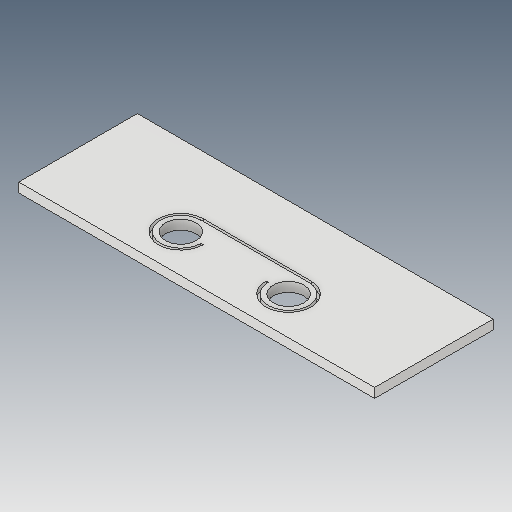
# Autodesk Inventor part: 2ureactor TorusTapa1
Saved by Autodesk Inventor 2018 (Build 220112000, 112)
## iProperties
Created: 2018-10-26
Part Number: 2ureactor TorusTapa1
Material: PPS Plastic
Document SubType Name: Modeling
Designer: mj.noguera10
Density: 1.637 g/cm^3
Appearance: Smooth - White
Author: mj.noguera10
Autodesk Inventor part; units mm, degrees
ref_plane "YZ Plane" through (0, 0, 0) normal (1, 0, 0) x (0, 1, 0)
ref_plane "XZ Plane" through (0, 0, 0) normal (0, 1, 0) x (-1, 0, 0)
ref_plane "XY Plane" through (0, 0, 0) normal (0, 0, 1) x (1, 0, 0)
sketch "Sombreado_1" plane through (0, 0, 0) normal (0, 0, 1) x (1, 0, 0)
  point P0 (0, 0)
sketch "Sombreado_2" plane through (0, 0, 0) normal (0, 0, 1) x (1, 0, 0)
  point P0 (0, 0)
sketch "Sombreado_3" plane through (0, 0, 0) normal (0, 0, 1) x (1, 0, 0)
  point P0 (0, 0)
sketch "Boceto1" plane through (0, 0, 0) normal (0, 1, 0) x (-1, 0, 0)
  line L0 (30.3882, 1.25) -> (30.8882, 1.25)
  line L1 (0, -6.75) -> (75, -6.75)
  line L2 (75, -6.75) -> (75, 18.25)
  line L3 (75, 18.25) -> (0, 18.25)
  line L4 (0, 18.25) -> (0, -6.75)
  arc A0 (21.3882, 1.25) -> (30.8882, 1.25) centre (26.1382, 1.25) ccw
  arc A1 (21.8882, 1.25) -> (30.3882, 1.25) centre (26.1382, 1.25) ccw
  line L5 (21.3882, 1.25) -> (21.8882, 1.25)
  line L6 (1.8, 2.5) -> (5.3, 2.5)
  line L7 (1.8, 2.5) -> (1.8, 3)
  line L8 (1.8, 3) -> (1, 3)
  line L9 (1, 3) -> (1, 2.5)
  line L10 (1, 0) -> (0, 0)
  line L11 (1, 0) -> (1, -0.5)
  line L12 (1, -0.5) -> (1.8, -0.5)
  line L13 (1.8, -0.5) -> (1.8, 0)
  line L14 (5.3, 0) -> (1.8, 0)
  line L15 (0, 2.5) -> (1, 2.5)
  line L16 (1.8, 11.5) -> (5.3, 11.5)
  line L17 (5.3, 9) -> (1.8, 9)
  line L18 (1, 9) -> (0, 9)
  line L19 (0, 11.5) -> (1, 11.5)
  line L20 (1.8, 11.5) -> (1.8, 12)
  line L21 (1.8, 12) -> (1, 12)
  line L22 (1, 12) -> (1, 11.5)
  line L23 (1, 9) -> (1, 8.5)
  line L24 (1, 8.5) -> (1.8, 8.5)
  line L25 (1.8, 8.5) -> (1.8, 9)
  line L26 (44.6082, 1.25) -> (44.1082, 1.25)
  arc A2 (44.1082, 1.25) -> (53.6082, 1.25) centre (48.8582, 1.25) ccw
  arc A3 (44.6082, 1.25) -> (53.1082, 1.25) centre (48.8582, 1.25) ccw
  line L27 (53.6082, 1.25) -> (53.1082, 1.25)
  line L28 (73.1964, 2.5) -> (69.6964, 2.5)
  line L29 (69.6964, 0) -> (73.1964, 0)
  line L30 (73.9964, 0) -> (74.9964, 0)
  line L31 (74.9964, 2.5) -> (73.9964, 2.5)
  line L32 (73.1964, 2.5) -> (73.1964, 3)
  line L33 (73.1964, 3) -> (73.9964, 3)
  line L34 (73.9964, 3) -> (73.9964, 2.5)
  line L35 (73.9964, 0) -> (73.9964, -0.5)
  line L36 (73.9964, -0.5) -> (73.1964, -0.5)
  line L37 (73.1964, -0.5) -> (73.1964, 0)
  line L38 (73.1964, 11.5) -> (69.6964, 11.5)
  line L39 (69.6964, 9) -> (73.1964, 9)
  line L40 (73.9964, 9) -> (74.9964, 9)
  line L41 (74.9964, 11.5) -> (73.9964, 11.5)
  line L42 (73.1964, 11.5) -> (73.1964, 12)
  line L43 (73.1964, 12) -> (73.9964, 12)
  line L44 (73.9964, 12) -> (73.9964, 11.5)
  line L45 (73.9964, 9) -> (73.9964, 8.5)
  line L46 (73.9964, 8.5) -> (73.1964, 8.5)
  line L47 (73.1964, 8.5) -> (73.1964, 9)
  line L48 (75, 18.25) -> (75, 43.25)
  line L49 (75, 43.25) -> (0, 43.25)
  line L50 (0, 43.25) -> (0, 18.25)
  line L51 (5.3, 11.5) -> (5.3, 9)
  line L52 (5.3, 2.5) -> (5.3, 0)
  line L53 (69.6964, 11.5) -> (69.6964, 9)
  line L54 (69.6964, 2.5) -> (69.6964, 0)
  circle A4 centre (26.1382, 1.25) radius 3.25
  circle A5 centre (48.8582, 1.25) radius 3.25
  circle A6 centre (26.1382, 26.25) radius 3.25
  circle A7 centre (48.8582, 26.25) radius 3.25
  line L55 (75, 43.25) -> (75, 68.25)
  line L56 (75, 68.25) -> (0, 68.25)
  line L57 (0, 68.25) -> (0, 43.25)
  circle A8 centre (26.1382, 51.25) radius 3.25
  circle A9 centre (48.8582, 51.25) radius 3.25
  point P0 (0, 0)
  constraints: 116 end point, 10 centre point, 8 point on circle
sketch "Boceto3" plane through (0, 0, 0) normal (0, 1, 0) x (-1, 0, 0)
  line L0 (0, 0) -> (-75, 0)
  line L1 (-75, 0) -> (-75, -25)
  line L2 (-75, -25) -> (0, -25)
  line L3 (0, -25) -> (0, 0)
  line L4 (0, 0) -> (-75, 0)
  line L5 (-75, 0) -> (-75, -25)
  line L6 (-75, -25) -> (0, -25)
  line L7 (0, -25) -> (0, 0)
  dimension "d4" = 75
  dimension "d5" = 25
  dimension "d6" = 75
  dimension "d7" = 25
  constraints: 16 end point, 4 parallel, 2 horizontal, 2 perpendicular
  measures "d4" distance of L2.end L1.end
  measures "d5" distance of L1.end L1.start
  measures "d6" distance of L6.end L5.end
  measures "d7" distance of L5.end L5.start
extrude "Extrusión1" add sketch "Boceto3" along normal blind 2
sketch "Boceto4" plane through (0, 2, 0) normal (0, 1, 0) x (1, 0, 0)
  circle A0 centre (26.1418, 8) radius 3.25
  line L0 (0, 0) -> (75, 0) projected
  line L1 (75, 25) -> (0, 25) projected
  circle A1 centre (48.8582, 8) radius 3.25
  constraints: 2 centre point
extrude "Extrusión2" cut sketch "Boceto4" against normal blind 2
sketch "Boceto5" plane through (0, 2, 0) normal (0, 1, 0) x (1, 0, 0)
  line L0 (30.8908, 8) -> (30.3928, 8)
  line L1 (44.1092, 8) -> (44.6072, 8)
  arc A0 (44.6072, 8) -> (48.8582, 12.251) centre (48.8582, 8) ccw
  arc A1 (44.1092, 8) -> (48.8582, 12.749) centre (48.8582, 8) ccw
  arc A2 (26.1418, 12.251) -> (30.3928, 8) centre (26.1418, 8) ccw
  arc A3 (26.1418, 12.749) -> (30.8908, 8) centre (26.1418, 8) ccw
  line L2 (26.1418, 12.251) -> (48.8582, 12.251)
  line L3 (26.1418, 12.749) -> (48.8582, 12.749)
  point P0 (0, 0)
  constraints: 9 point on circle, 8 end point, 4 centre point, 2 coincident, 2 horizontal, 1 tangent
extrude "Extrusión3" cut sketch "Boceto5" against normal blind 1
